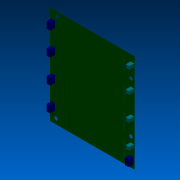
# Autodesk Inventor part: MotorDriver Main Board_CPY
Saved by Autodesk Inventor 2013 (Build 170138000, 138)
## iProperties
Created: 2014-11-03
Part Number: MotorDriver Main Board_CPY
Material: Generic
Document SubType Name: Modeling
Designer: Jeramy
Density: 1 g/cm^3
Author: Jeramy
Autodesk Inventor part; units mm, degrees
ref_plane "YZ Plane" through (0, 0, 0) normal (1, 0, 0) x (0, 1, 0)
ref_plane "XZ Plane" through (0, 0, 0) normal (0, 1, 0) x (-1, 0, 0)
ref_plane "XY Plane" through (0, 0, 0) normal (0, 0, 1) x (1, 0, 0)
sketch "Sketch1" plane through (0, 0, 0) normal (0, 0, 1) x (1, 0, 0)
  line L0 (215.9, 224.8) -> (349.3, 224.8)
  line L1 (349.3, 224.8) -> (349.3, 379.7)
  line L2 (349.3, 379.7) -> (215.9, 379.7)
  line L3 (215.9, 379.7) -> (215.9, 224.8)
  arc A0 (224.8, 373.4) -> (229.9, 372.1) centre (227.35, 372.75) ccw
  arc A1 (229.9, 372.1) -> (224.8, 373.4) centre (227.35, 372.75) ccw
  arc A2 (344.2, 349.3) -> (342.9, 344.2) centre (343.55, 346.75) ccw
  arc A3 (342.9, 344.2) -> (344.2, 349.3) centre (343.55, 346.75) ccw
  arc A4 (223.5, 234.9) -> (227.3, 231.1) centre (225.4, 233) ccw
  arc A5 (227.3, 231.1) -> (223.5, 234.9) centre (225.4, 233) ccw
  arc A6 (345.4, 269.2) -> (341.6, 265.4) centre (343.5, 267.3) ccw
  arc A7 (341.6, 265.4) -> (345.4, 269.2) centre (343.5, 267.3) ccw
  circle A8 centre (221, 356.9) radius 0.5
  circle A9 centre (221, 359.4) radius 0.5
  circle A10 centre (221, 361.9) radius 0.5
  circle A11 centre (221, 364.5) radius 0.5
  circle A12 centre (221, 320) radius 0.5
  circle A13 centre (221, 322.6) radius 0.5
  circle A14 centre (221, 325.1) radius 0.5
  circle A15 centre (221, 327.7) radius 0.5
  circle A16 centre (221, 281.9) radius 0.5
  circle A17 centre (221, 284.5) radius 0.5
  circle A18 centre (221, 287) radius 0.5
  circle A19 centre (221, 289.6) radius 0.5
  circle A20 centre (221, 243.8) radius 0.5
  circle A21 centre (221, 246.4) radius 0.5
  circle A22 centre (221, 248.9) radius 0.5
  circle A23 centre (221, 251.5) radius 0.5
  circle A24 centre (345.4, 368.3) radius 0.5
  circle A25 centre (345.4, 365.8) radius 0.5
  circle A26 centre (345.4, 334) radius 0.5
  circle A27 centre (345.4, 331.5) radius 0.5
  circle A28 centre (345.4, 295.9) radius 0.5
  circle A29 centre (345.4, 293.4) radius 0.5
  circle A30 centre (345.4, 257.8) radius 0.5
  circle A31 centre (345.4, 255.3) radius 0.5
  circle A32 centre (344.2, 240) radius 0.5
  circle A33 centre (344.2, 237.5) radius 0.5
  circle A34 centre (344.2, 234.9) radius 0.5
  circle A35 centre (344.2, 232.4) radius 0.5
  circle A36 centre (331.5, 256.5) radius 0.4
  circle A37 centre (334, 256.5) radius 0.4
  circle A38 centre (241.3, 252.7) radius 0.4
  circle A39 centre (241.3, 255.3) radius 0.4
  circle A40 centre (241.3, 247.7) radius 0.4
  circle A41 centre (241.3, 250.2) radius 0.4
  circle A42 centre (241.3, 245.1) radius 0.4
  circle A43 centre (241.3, 242.6) radius 0.4
  circle A44 centre (241.3, 237.5) radius 0.4
  circle A45 centre (241.3, 240) radius 0.4
  circle A46 centre (241.3, 232.4) radius 0.4
  circle A47 centre (241.3, 234.9) radius 0.4
  circle A48 centre (331.5, 251.5) radius 0.4
  circle A49 centre (331.5, 254) radius 0.4
  circle A50 centre (334, 251.5) radius 0.4
  circle A51 centre (334, 254) radius 0.4
  circle A52 centre (331.5, 246.4) radius 0.4
  circle A53 centre (331.5, 248.9) radius 0.4
  circle A54 centre (334, 246.4) radius 0.4
  circle A55 centre (334, 248.9) radius 0.4
  circle A56 centre (331.5, 241.3) radius 0.4
  circle A57 centre (331.5, 243.8) radius 0.4
  circle A58 centre (334, 243.8) radius 0.4
  circle A59 centre (334, 241.3) radius 0.4
  circle A60 centre (331.5, 238.8) radius 0.4
  circle A61 centre (331.5, 236.2) radius 0.4
  circle A62 centre (334, 238.8) radius 0.4
  circle A63 centre (334, 236.2) radius 0.4
  circle A64 centre (331.5, 233.7) radius 0.4
  circle A65 centre (334, 233.7) radius 0.4
  circle A66 centre (331.5, 294.6) radius 0.4
  circle A67 centre (334, 294.6) radius 0.4
  circle A68 centre (241.3, 290.8) radius 0.4
  circle A69 centre (241.3, 293.4) radius 0.4
  circle A70 centre (241.3, 285.8) radius 0.4
  circle A71 centre (241.3, 288.3) radius 0.4
  circle A72 centre (241.3, 283.2) radius 0.4
  circle A73 centre (241.3, 280.7) radius 0.4
  circle A74 centre (241.3, 275.6) radius 0.4
  circle A75 centre (241.3, 278.1) radius 0.4
  circle A76 centre (241.3, 270.5) radius 0.4
  circle A77 centre (241.3, 273.1) radius 0.4
  circle A78 centre (331.5, 289.6) radius 0.4
  circle A79 centre (331.5, 292.1) radius 0.4
  circle A80 centre (334, 289.6) radius 0.4
  circle A81 centre (334, 292.1) radius 0.4
  circle A82 centre (331.5, 284.5) radius 0.4
  circle A83 centre (331.5, 287) radius 0.4
  circle A84 centre (334, 284.5) radius 0.4
  circle A85 centre (334, 287) radius 0.4
  circle A86 centre (331.5, 279.4) radius 0.4
  circle A87 centre (331.5, 281.9) radius 0.4
  circle A88 centre (334, 281.9) radius 0.4
  circle A89 centre (334, 279.4) radius 0.4
  circle A90 centre (331.5, 276.9) radius 0.4
  circle A91 centre (331.5, 274.3) radius 0.4
  circle A92 centre (334, 276.9) radius 0.4
  circle A93 centre (334, 274.3) radius 0.4
  circle A94 centre (331.5, 271.8) radius 0.4
  circle A95 centre (334, 271.8) radius 0.4
  circle A96 centre (331.5, 332.7) radius 0.4
  circle A97 centre (334, 332.7) radius 0.4
  circle A98 centre (241.3, 328.9) radius 0.4
  circle A99 centre (241.3, 331.5) radius 0.4
  circle A100 centre (241.3, 323.9) radius 0.4
  circle A101 centre (241.3, 326.4) radius 0.4
  circle A102 centre (241.3, 321.3) radius 0.4
  circle A103 centre (241.3, 318.8) radius 0.4
  circle A104 centre (241.3, 313.7) radius 0.4
  circle A105 centre (241.3, 316.2) radius 0.4
  circle A106 centre (241.3, 308.6) radius 0.4
  circle A107 centre (241.3, 311.1) radius 0.4
  circle A108 centre (331.5, 327.7) radius 0.4
  circle A109 centre (331.5, 330.2) radius 0.4
  circle A110 centre (334, 327.7) radius 0.4
  circle A111 centre (334, 330.2) radius 0.4
  circle A112 centre (331.5, 322.6) radius 0.4
  circle A113 centre (331.5, 325.1) radius 0.4
  circle A114 centre (334, 322.6) radius 0.4
  circle A115 centre (334, 325.1) radius 0.4
  circle A116 centre (331.5, 317.5) radius 0.4
  circle A117 centre (331.5, 320) radius 0.4
  circle A118 centre (334, 320) radius 0.4
  circle A119 centre (334, 317.5) radius 0.4
  circle A120 centre (331.5, 315) radius 0.4
  circle A121 centre (331.5, 312.4) radius 0.4
  circle A122 centre (334, 315) radius 0.4
  circle A123 centre (334, 312.4) radius 0.4
  circle A124 centre (331.5, 309.9) radius 0.4
  circle A125 centre (334, 309.9) radius 0.4
  circle A126 centre (331.5, 370.8) radius 0.4
  circle A127 centre (334, 370.8) radius 0.4
  circle A128 centre (241.3, 367) radius 0.4
  circle A129 centre (241.3, 369.6) radius 0.4
  circle A130 centre (241.3, 361.9) radius 0.4
  circle A131 centre (241.3, 364.5) radius 0.4
  circle A132 centre (241.3, 359.4) radius 0.4
  circle A133 centre (241.3, 356.9) radius 0.4
  circle A134 centre (241.3, 351.8) radius 0.4
  circle A135 centre (241.3, 354.3) radius 0.4
  circle A136 centre (241.3, 346.7) radius 0.4
  circle A137 centre (241.3, 349.3) radius 0.4
  circle A138 centre (331.5, 365.8) radius 0.4
  circle A139 centre (331.5, 368.3) radius 0.4
  circle A140 centre (334, 365.8) radius 0.4
  circle A141 centre (334, 368.3) radius 0.4
  circle A142 centre (331.5, 360.7) radius 0.4
  circle A143 centre (331.5, 363.2) radius 0.4
  circle A144 centre (334, 360.7) radius 0.4
  circle A145 centre (334, 363.2) radius 0.4
  circle A146 centre (331.5, 355.6) radius 0.4
  circle A147 centre (331.5, 358.1) radius 0.4
  circle A148 centre (334, 358.1) radius 0.4
  circle A149 centre (334, 355.6) radius 0.4
  circle A150 centre (331.5, 353.1) radius 0.4
  circle A151 centre (331.5, 350.5) radius 0.4
  circle A152 centre (334, 353.1) radius 0.4
  circle A153 centre (334, 350.5) radius 0.4
  circle A154 centre (331.5, 348) radius 0.4
  circle A155 centre (334, 348) radius 0.4
  constraints: 156 centre point, 16 point on circle, 8 end point
extrude "MotorDriver Main Board_Outline" add sketch "Sketch1" along normal blind 0.01
sketch "MOLEX-1X4, M04POLAR_1" plane through (0, 0, 0.01) normal (0, 0, 1) x (1, 0, 0)
  line L0 (223.5, 355.6) -> (218, 355.6)
  line L1 (218, 355.6) -> (218, 365.8)
  line L2 (218, 365.8) -> (223.5, 365.8)
  line L3 (223.5, 365.8) -> (223.5, 355.6)
  constraints: 8 end point
extrude "JP1_2" add sketch "MOLEX-1X4, M04POLAR_1" along normal blind 7.5
sketch "MOLEX-1X4, M04POLAR_3" plane through (0, 0, 0.01) normal (0, 0, 1) x (1, 0, 0)
  line L0 (223.5, 318.7) -> (218, 318.7)
  line L1 (218, 318.7) -> (218, 328.9)
  line L2 (218, 328.9) -> (223.5, 328.9)
  line L3 (223.5, 328.9) -> (223.5, 318.7)
  constraints: 8 end point
extrude "JP2_4" add sketch "MOLEX-1X4, M04POLAR_3" along normal blind 7.5
sketch "MOLEX-1X4, M04POLAR_5" plane through (0, 0, 0.01) normal (0, 0, 1) x (1, 0, 0)
  line L0 (223.5, 280.6) -> (218, 280.6)
  line L1 (218, 280.6) -> (218, 290.8)
  line L2 (218, 290.8) -> (223.5, 290.8)
  line L3 (223.5, 290.8) -> (223.5, 280.6)
  constraints: 8 end point
extrude "JP3_6" add sketch "MOLEX-1X4, M04POLAR_5" along normal blind 7.5
sketch "MOLEX-1X4, M04POLAR_7" plane through (0, 0, 0.01) normal (0, 0, 1) x (1, 0, 0)
  line L0 (223.5, 242.5) -> (218, 242.5)
  line L1 (218, 242.5) -> (218, 252.7)
  line L2 (218, 252.7) -> (223.5, 252.7)
  line L3 (223.5, 252.7) -> (223.5, 242.5)
  constraints: 8 end point
extrude "JP4_8" add sketch "MOLEX-1X4, M04POLAR_7" along normal blind 7.5
sketch "MOLEX-1X2, M02POLAR_9" plane through (0, 0, 0.01) normal (0, 0, 1) x (1, 0, 0)
  line L0 (342.9, 369.6) -> (348.4, 369.6)
  line L1 (348.4, 369.6) -> (348.4, 364.5)
  line L2 (348.4, 364.5) -> (342.9, 364.5)
  line L3 (342.9, 364.5) -> (342.9, 369.6)
  constraints: 8 end point
extrude "JP5_10" add sketch "MOLEX-1X2, M02POLAR_9" along normal blind 7.5
sketch "MOLEX-1X2, M02POLAR_11" plane through (0, 0, 0.01) normal (0, 0, 1) x (1, 0, 0)
  line L0 (342.9, 335.3) -> (348.4, 335.3)
  line L1 (348.4, 335.3) -> (348.4, 330.2)
  line L2 (348.4, 330.2) -> (342.9, 330.2)
  line L3 (342.9, 330.2) -> (342.9, 335.3)
  constraints: 8 end point
extrude "JP6_12" add sketch "MOLEX-1X2, M02POLAR_11" along normal blind 7.5
sketch "MOLEX-1X2, M02POLAR_13" plane through (0, 0, 0.01) normal (0, 0, 1) x (1, 0, 0)
  line L0 (342.9, 297.2) -> (348.4, 297.2)
  line L1 (348.4, 297.2) -> (348.4, 292.1)
  line L2 (348.4, 292.1) -> (342.9, 292.1)
  line L3 (342.9, 292.1) -> (342.9, 297.2)
  constraints: 8 end point
extrude "JP7_14" add sketch "MOLEX-1X2, M02POLAR_13" along normal blind 7.5
sketch "MOLEX-1X2, M02POLAR_15" plane through (0, 0, 0.01) normal (0, 0, 1) x (1, 0, 0)
  line L0 (342.9, 259.1) -> (348.4, 259.1)
  line L1 (348.4, 259.1) -> (348.4, 254)
  line L2 (348.4, 254) -> (342.9, 254)
  line L3 (342.9, 254) -> (342.9, 259.1)
  constraints: 8 end point
extrude "JP8_16" add sketch "MOLEX-1X2, M02POLAR_15" along normal blind 7.5
sketch "MOLEX-1X4, M04POLAR_17" plane through (0, 0, 0.01) normal (0, 0, 1) x (1, 0, 0)
  line L0 (341.7, 241.3) -> (347.2, 241.3)
  line L1 (347.2, 241.3) -> (347.2, 231.1)
  line L2 (347.2, 231.1) -> (341.7, 231.1)
  line L3 (341.7, 231.1) -> (341.7, 241.3)
  constraints: 8 end point
extrude "JP9_18" add sketch "MOLEX-1X4, M04POLAR_17" along normal blind 7.5
body "Solid1"
